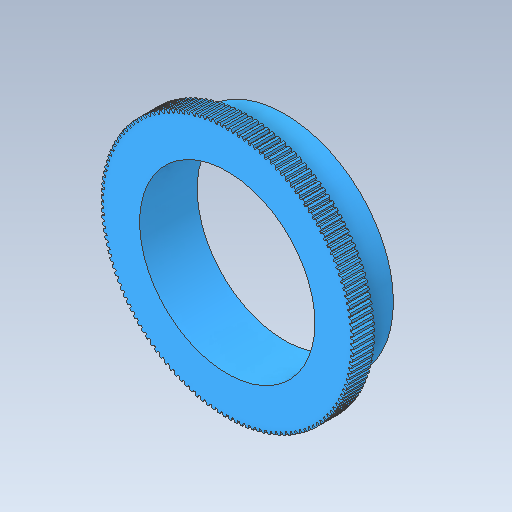
# Autodesk Inventor part: タミヤダンパー4
Saved by Autodesk Inventor 2020 (Build 240168000, 168)
## iProperties
Part Number: タミヤダンパー4
Material: 一般
Document SubType Name: Modeling
Designer: 雪村
Density: 1 g/cm^3
Appearance: 既定
Mass: 0.362407 g
Surface Area: 6.8095 cm^2
Volume: 0.362407 cm^3
Author: 雪村
Autodesk Inventor part; units mm, degrees
ref_plane "YZ Plane" through (0, 0, 0) normal (1, 0, 0) x (0, 1, 0)
ref_plane "XZ Plane" through (0, 0, 0) normal (0, 1, 0) x (-1, 0, 0)
ref_plane "XY Plane" through (0, 0, 0) normal (0, 0, 1) x (1, 0, 0)
sketch "スケッチ1" plane through (0, 0, 0) normal (0, 0, 1) x (1, 0, 0)
  circle A0 centre (0, 0) radius 7.75
  dimension "d0" = 15.5
  constraints: 1 centre point, 1 coincident
  measures "d0" diameter of A0
extrude "押し出し1" add sketch "スケッチ1" along normal blind 2.6
sketch "スケッチ2" plane through (0, 0, 2.6) normal (0, 0, 1) x (1, 0, 0)
  circle A0 centre (0, 0) radius 9
  dimension "d3" = 18
  constraints: 1 centre point, 1 coincident
  measures "d3" diameter of A0
extrude "押し出し2" add sketch "スケッチ2" along normal blind 1.5
sketch "スケッチ3" plane through (0, 0, 4.1) normal (0, 0, 1) x (1, 0, 0)
  circle A0 centre (0, 0) radius 6.25
  dimension "d6" = 12.5
  constraints: 1 centre point, 1 coincident
  measures "d6" diameter of A0
extrude "押し出し3" cut sketch "スケッチ3" against normal through all
sketch "スケッチ4" plane through (0, 0, 4.1) normal (0, 0, 1) x (1, 0, 0)
  arc A0 (-0.1214, -8.9992) -> (0.1214, -8.9992) centre (0, 0) ccw
  arc A1 (-0.05, -8.8124) -> (0.05, -8.8124) centre (0, 0) ccw
  line L0 (0.1214, -8.9992) -> (0.05, -8.8124)
  line L1 (-0.05, -8.8124) -> (-0.1214, -8.9992)
  line L2 (0, -8.8125) -> (0, 0)
  line L3 (0.525, -8.9847) -> (0.4453, -8.8012)
  arc A2 (0.2825, -8.9956) -> (0.525, -8.9847) centre (0, 0) ccw
  line L4 (0.3454, -8.8057) -> (0.2825, -8.9956)
  arc A3 (0.3454, -8.8057) -> (0.4453, -8.8012) centre (0, 0) ccw
  line L5 (0.9276, -8.9521) -> (0.8397, -8.7724)
  arc A4 (0.6858, -8.9738) -> (0.9276, -8.9521) centre (0, 0) ccw
  line L6 (0.7401, -8.7814) -> (0.6858, -8.9738)
  arc A5 (0.7401, -8.7814) -> (0.8397, -8.7724) centre (0, 0) ccw
  line L7 (1.3283, -8.9014) -> (1.2325, -8.7259)
  arc A6 (1.0877, -8.934) -> (1.3283, -8.9014) centre (0, 0) ccw
  line L8 (1.1334, -8.7393) -> (1.0877, -8.934)
  arc A7 (1.1334, -8.7393) -> (1.2325, -8.7259) centre (0, 0) ccw
  line L9 (1.7263, -8.8329) -> (1.6227, -8.6618)
  arc A8 (1.4874, -8.8762) -> (1.7263, -8.8329) centre (0, 0) ccw
  line L10 (1.5243, -8.6797) -> (1.4874, -8.8762)
  arc A9 (1.5243, -8.6797) -> (1.6227, -8.6618) centre (0, 0) ccw
  line L11 (2.1209, -8.7465) -> (2.0097, -8.5803)
  arc A10 (1.8842, -8.8006) -> (2.1209, -8.7465) centre (0, 0) ccw
  line L12 (1.9122, -8.6025) -> (1.8842, -8.8006)
  arc A11 (1.9122, -8.6025) -> (2.0097, -8.5803) centre (0, 0) ccw
  line L13 (2.5111, -8.6426) -> (2.3926, -8.4815)
  arc A12 (2.2771, -8.7072) -> (2.5111, -8.6426) centre (0, 0) ccw
  line L14 (2.2962, -8.5081) -> (2.2771, -8.7072)
  arc A13 (2.2962, -8.5081) -> (2.3926, -8.4815) centre (0, 0) ccw
  line L15 (2.8964, -8.5212) -> (2.7707, -8.3656)
  arc A14 (2.6654, -8.5962) -> (2.8964, -8.5212) centre (0, 0) ccw
  line L16 (2.6756, -8.3965) -> (2.6654, -8.5962)
  arc A15 (2.6756, -8.3965) -> (2.7707, -8.3656) centre (0, 0) ccw
  line L17 (3.2757, -8.3827) -> (3.1433, -8.2329)
  arc A16 (3.0484, -8.468) -> (3.2757, -8.3827) centre (0, 0) ccw
  line L18 (3.0496, -8.268) -> (3.0484, -8.468)
  arc A17 (3.0496, -8.268) -> (3.1433, -8.2329) centre (0, 0) ccw
  line L19 (3.6485, -8.2273) -> (3.5095, -8.0836)
  arc A18 (3.4253, -8.3227) -> (3.6485, -8.2273) centre (0, 0) ccw
  line L20 (3.4175, -8.1229) -> (3.4253, -8.3227)
  arc A19 (3.4175, -8.1229) -> (3.5095, -8.0836) centre (0, 0) ccw
  line L21 (4.014, -8.0553) -> (3.8686, -7.918)
  arc A20 (3.7952, -8.1607) -> (4.014, -8.0553) centre (0, 0) ccw
  line L22 (3.7785, -7.9614) -> (3.7952, -8.1607)
  arc A21 (3.7785, -7.9614) -> (3.8686, -7.918) centre (0, 0) ccw
  line L23 (4.3713, -7.8671) -> (4.2199, -7.7364)
  arc A22 (4.1575, -7.9822) -> (4.3713, -7.8671) centre (0, 0) ccw
  line L24 (4.1319, -7.7838) -> (4.1575, -7.9822)
  arc A23 (4.1319, -7.7838) -> (4.2199, -7.7364) centre (0, 0) ccw
  line L25 (4.7199, -7.6631) -> (4.5628, -7.5393)
  arc A24 (4.5115, -7.7876) -> (4.7199, -7.6631) centre (0, 0) ccw
  line L26 (4.4769, -7.5906) -> (4.5115, -7.7876)
  arc A25 (4.4769, -7.5906) -> (4.5628, -7.5393) centre (0, 0) ccw
  line L27 (5.0589, -7.4436) -> (4.8964, -7.327)
  arc A26 (4.8563, -7.5774) -> (5.0589, -7.4436) centre (0, 0) ccw
  line L28 (4.813, -7.3821) -> (4.8563, -7.5774)
  arc A27 (4.813, -7.3821) -> (4.8964, -7.327) centre (0, 0) ccw
  line L29 (5.3878, -7.2091) -> (5.2202, -7.1)
  arc A28 (5.1914, -7.3518) -> (5.3878, -7.2091) centre (0, 0) ccw
  line L30 (5.1393, -7.1587) -> (5.1914, -7.3518)
  arc A29 (5.1393, -7.1587) -> (5.2202, -7.1) centre (0, 0) ccw
  line L31 (5.7058, -6.9602) -> (5.5335, -6.8586)
  arc A30 (5.516, -7.1115) -> (5.7058, -6.9602) centre (0, 0) ccw
  line L32 (5.4553, -6.921) -> (5.516, -7.1115)
  arc A31 (5.4553, -6.921) -> (5.5335, -6.8586) centre (0, 0) ccw
  line L33 (6.0123, -6.6972) -> (5.8356, -6.6034)
  arc A32 (5.8295, -6.8569) -> (6.0123, -6.6972) centre (0, 0) ccw
  line L34 (5.7603, -6.6692) -> (5.8295, -6.8569)
  arc A33 (5.7603, -6.6692) -> (5.8356, -6.6034) centre (0, 0) ccw
  line L35 (6.3067, -6.4207) -> (6.126, -6.335)
  arc A34 (6.1313, -6.5885) -> (6.3067, -6.4207) centre (0, 0) ccw
  line L36 (6.0538, -6.4041) -> (6.1313, -6.5885)
  arc A35 (6.0538, -6.4041) -> (6.126, -6.335) centre (0, 0) ccw
  line L37 (6.5885, -6.1313) -> (6.4041, -6.0538)
  arc A36 (6.4207, -6.3067) -> (6.5885, -6.1313) centre (0, 0) ccw
  line L38 (6.335, -6.126) -> (6.4207, -6.3067)
  arc A37 (6.335, -6.126) -> (6.4041, -6.0538) centre (0, 0) ccw
  line L39 (6.8569, -5.8295) -> (6.6692, -5.7603)
  arc A38 (6.6972, -6.0123) -> (6.8569, -5.8295) centre (0, 0) ccw
  line L40 (6.6034, -5.8356) -> (6.6972, -6.0123)
  arc A39 (6.6034, -5.8356) -> (6.6692, -5.7603) centre (0, 0) ccw
  line L41 (7.1115, -5.516) -> (6.921, -5.4553)
  arc A40 (6.9602, -5.7058) -> (7.1115, -5.516) centre (0, 0) ccw
  line L42 (6.8586, -5.5335) -> (6.9602, -5.7058)
  arc A41 (6.8586, -5.5335) -> (6.921, -5.4553) centre (0, 0) ccw
  line L43 (7.3518, -5.1914) -> (7.1587, -5.1393)
  arc A42 (7.2091, -5.3878) -> (7.3518, -5.1914) centre (0, 0) ccw
  line L44 (7.1, -5.2202) -> (7.2091, -5.3878)
  arc A43 (7.1, -5.2202) -> (7.1587, -5.1393) centre (0, 0) ccw
  line L45 (7.5774, -4.8563) -> (7.3821, -4.813)
  arc A44 (7.4436, -5.0589) -> (7.5774, -4.8563) centre (0, 0) ccw
  line L46 (7.327, -4.8964) -> (7.4436, -5.0589)
  arc A45 (7.327, -4.8964) -> (7.3821, -4.813) centre (0, 0) ccw
  line L47 (7.7876, -4.5115) -> (7.5906, -4.4769)
  arc A46 (7.6631, -4.7199) -> (7.7876, -4.5115) centre (0, 0) ccw
  line L48 (7.5393, -4.5628) -> (7.6631, -4.7199)
  arc A47 (7.5393, -4.5628) -> (7.5906, -4.4769) centre (0, 0) ccw
  line L49 (7.9822, -4.1575) -> (7.7838, -4.1319)
  arc A48 (7.8671, -4.3713) -> (7.9822, -4.1575) centre (0, 0) ccw
  line L50 (7.7364, -4.2199) -> (7.8671, -4.3713)
  arc A49 (7.7364, -4.2199) -> (7.7838, -4.1319) centre (0, 0) ccw
  line L51 (8.1607, -3.7952) -> (7.9614, -3.7785)
  arc A50 (8.0553, -4.014) -> (8.1607, -3.7952) centre (0, 0) ccw
  line L52 (7.918, -3.8686) -> (8.0553, -4.014)
  arc A51 (7.918, -3.8686) -> (7.9614, -3.7785) centre (0, 0) ccw
  line L53 (8.3227, -3.4253) -> (8.1229, -3.4175)
  arc A52 (8.2273, -3.6485) -> (8.3227, -3.4253) centre (0, 0) ccw
  line L54 (8.0836, -3.5095) -> (8.2273, -3.6485)
  arc A53 (8.0836, -3.5095) -> (8.1229, -3.4175) centre (0, 0) ccw
  line L55 (8.468, -3.0484) -> (8.268, -3.0496)
  arc A54 (8.3827, -3.2757) -> (8.468, -3.0484) centre (0, 0) ccw
  line L56 (8.2329, -3.1433) -> (8.3827, -3.2757)
  arc A55 (8.2329, -3.1433) -> (8.268, -3.0496) centre (0, 0) ccw
  line L57 (8.5962, -2.6654) -> (8.3965, -2.6756)
  arc A56 (8.5212, -2.8964) -> (8.5962, -2.6654) centre (0, 0) ccw
  line L58 (8.3656, -2.7707) -> (8.5212, -2.8964)
  arc A57 (8.3656, -2.7707) -> (8.3965, -2.6756) centre (0, 0) ccw
  line L59 (8.7072, -2.2771) -> (8.5081, -2.2962)
  arc A58 (8.6426, -2.5111) -> (8.7072, -2.2771) centre (0, 0) ccw
  line L60 (8.4815, -2.3926) -> (8.6426, -2.5111)
  arc A59 (8.4815, -2.3926) -> (8.5081, -2.2962) centre (0, 0) ccw
  line L61 (8.8006, -1.8842) -> (8.6025, -1.9122)
  arc A60 (8.7465, -2.1209) -> (8.8006, -1.8842) centre (0, 0) ccw
  line L62 (8.5803, -2.0097) -> (8.7465, -2.1209)
  arc A61 (8.5803, -2.0097) -> (8.6025, -1.9122) centre (0, 0) ccw
  line L63 (8.8762, -1.4874) -> (8.6797, -1.5243)
  arc A62 (8.8329, -1.7263) -> (8.8762, -1.4874) centre (0, 0) ccw
  line L64 (8.6618, -1.6227) -> (8.8329, -1.7263)
  arc A63 (8.6618, -1.6227) -> (8.6797, -1.5243) centre (0, 0) ccw
  line L65 (8.934, -1.0877) -> (8.7393, -1.1334)
  arc A64 (8.9014, -1.3283) -> (8.934, -1.0877) centre (0, 0) ccw
  line L66 (8.7259, -1.2325) -> (8.9014, -1.3283)
  arc A65 (8.7259, -1.2325) -> (8.7393, -1.1334) centre (0, 0) ccw
  line L67 (8.9738, -0.6858) -> (8.7814, -0.7401)
  arc A66 (8.9521, -0.9276) -> (8.9738, -0.6858) centre (0, 0) ccw
  line L68 (8.7724, -0.8397) -> (8.9521, -0.9276)
  arc A67 (8.7724, -0.8397) -> (8.7814, -0.7401) centre (0, 0) ccw
  line L69 (8.9956, -0.2825) -> (8.8057, -0.3454)
  arc A68 (8.9847, -0.525) -> (8.9956, -0.2825) centre (0, 0) ccw
  line L70 (8.8012, -0.4453) -> (8.9847, -0.525)
  arc A69 (8.8012, -0.4453) -> (8.8057, -0.3454) centre (0, 0) ccw
  line L71 (8.9992, 0.1214) -> (8.8124, 0.05)
  arc A70 (8.9992, -0.1214) -> (8.9992, 0.1214) centre (0, 0) ccw
  line L72 (8.8124, -0.05) -> (8.9992, -0.1214)
  arc A71 (8.8124, -0.05) -> (8.8124, 0.05) centre (0, 0) ccw
  line L73 (8.9847, 0.525) -> (8.8012, 0.4453)
  arc A72 (8.9956, 0.2825) -> (8.9847, 0.525) centre (0, 0) ccw
  line L74 (8.8057, 0.3454) -> (8.9956, 0.2825)
  arc A73 (8.8057, 0.3454) -> (8.8012, 0.4453) centre (0, 0) ccw
  line L75 (8.9521, 0.9276) -> (8.7724, 0.8397)
  arc A74 (8.9738, 0.6858) -> (8.9521, 0.9276) centre (0, 0) ccw
  line L76 (8.7814, 0.7401) -> (8.9738, 0.6858)
  arc A75 (8.7814, 0.7401) -> (8.7724, 0.8397) centre (0, 0) ccw
  line L77 (8.9014, 1.3283) -> (8.7259, 1.2325)
  arc A76 (8.934, 1.0877) -> (8.9014, 1.3283) centre (0, 0) ccw
  line L78 (8.7393, 1.1334) -> (8.934, 1.0877)
  arc A77 (8.7393, 1.1334) -> (8.7259, 1.2325) centre (0, 0) ccw
  line L79 (8.8329, 1.7263) -> (8.6618, 1.6227)
  arc A78 (8.8762, 1.4874) -> (8.8329, 1.7263) centre (0, 0) ccw
  line L80 (8.6797, 1.5243) -> (8.8762, 1.4874)
  arc A79 (8.6797, 1.5243) -> (8.6618, 1.6227) centre (0, 0) ccw
  line L81 (8.7465, 2.1209) -> (8.5803, 2.0097)
  arc A80 (8.8006, 1.8842) -> (8.7465, 2.1209) centre (0, 0) ccw
  line L82 (8.6025, 1.9122) -> (8.8006, 1.8842)
  arc A81 (8.6025, 1.9122) -> (8.5803, 2.0097) centre (0, 0) ccw
  line L83 (8.6426, 2.5111) -> (8.4815, 2.3926)
  arc A82 (8.7072, 2.2771) -> (8.6426, 2.5111) centre (0, 0) ccw
  line L84 (8.5081, 2.2962) -> (8.7072, 2.2771)
  arc A83 (8.5081, 2.2962) -> (8.4815, 2.3926) centre (0, 0) ccw
  line L85 (8.5212, 2.8964) -> (8.3656, 2.7707)
  arc A84 (8.5962, 2.6654) -> (8.5212, 2.8964) centre (0, 0) ccw
  line L86 (8.3965, 2.6756) -> (8.5962, 2.6654)
  arc A85 (8.3965, 2.6756) -> (8.3656, 2.7707) centre (0, 0) ccw
  line L87 (8.3827, 3.2757) -> (8.2329, 3.1433)
  arc A86 (8.468, 3.0484) -> (8.3827, 3.2757) centre (0, 0) ccw
  line L88 (8.268, 3.0496) -> (8.468, 3.0484)
  arc A87 (8.268, 3.0496) -> (8.2329, 3.1433) centre (0, 0) ccw
  line L89 (8.2273, 3.6485) -> (8.0836, 3.5095)
  arc A88 (8.3227, 3.4253) -> (8.2273, 3.6485) centre (0, 0) ccw
  line L90 (8.1229, 3.4175) -> (8.3227, 3.4253)
  arc A89 (8.1229, 3.4175) -> (8.0836, 3.5095) centre (0, 0) ccw
  line L91 (8.0553, 4.014) -> (7.918, 3.8686)
  arc A90 (8.1607, 3.7952) -> (8.0553, 4.014) centre (0, 0) ccw
  line L92 (7.9614, 3.7785) -> (8.1607, 3.7952)
  arc A91 (7.9614, 3.7785) -> (7.918, 3.8686) centre (0, 0) ccw
  line L93 (7.8671, 4.3713) -> (7.7364, 4.2199)
  arc A92 (7.9822, 4.1575) -> (7.8671, 4.3713) centre (0, 0) ccw
  line L94 (7.7838, 4.1319) -> (7.9822, 4.1575)
  arc A93 (7.7838, 4.1319) -> (7.7364, 4.2199) centre (0, 0) ccw
  line L95 (7.6631, 4.7199) -> (7.5393, 4.5628)
  arc A94 (7.7876, 4.5115) -> (7.6631, 4.7199) centre (0, 0) ccw
  line L96 (7.5906, 4.4769) -> (7.7876, 4.5115)
  arc A95 (7.5906, 4.4769) -> (7.5393, 4.5628) centre (0, 0) ccw
  line L97 (7.4436, 5.0589) -> (7.327, 4.8964)
  arc A96 (7.5774, 4.8563) -> (7.4436, 5.0589) centre (0, 0) ccw
  line L98 (7.3821, 4.813) -> (7.5774, 4.8563)
  arc A97 (7.3821, 4.813) -> (7.327, 4.8964) centre (0, 0) ccw
  line L99 (7.2091, 5.3878) -> (7.1, 5.2202)
  arc A98 (7.3518, 5.1914) -> (7.2091, 5.3878) centre (0, 0) ccw
  line L100 (7.1587, 5.1393) -> (7.3518, 5.1914)
  arc A99 (7.1587, 5.1393) -> (7.1, 5.2202) centre (0, 0) ccw
  line L101 (6.9602, 5.7058) -> (6.8586, 5.5335)
  arc A100 (7.1115, 5.516) -> (6.9602, 5.7058) centre (0, 0) ccw
  line L102 (6.921, 5.4553) -> (7.1115, 5.516)
  arc A101 (6.921, 5.4553) -> (6.8586, 5.5335) centre (0, 0) ccw
  line L103 (6.6972, 6.0123) -> (6.6034, 5.8356)
  arc A102 (6.8569, 5.8295) -> (6.6972, 6.0123) centre (0, 0) ccw
  line L104 (6.6692, 5.7603) -> (6.8569, 5.8295)
  arc A103 (6.6692, 5.7603) -> (6.6034, 5.8356) centre (0, 0) ccw
  line L105 (6.4207, 6.3067) -> (6.335, 6.126)
  arc A104 (6.5885, 6.1313) -> (6.4207, 6.3067) centre (0, 0) ccw
  line L106 (6.4041, 6.0538) -> (6.5885, 6.1313)
  arc A105 (6.4041, 6.0538) -> (6.335, 6.126) centre (0, 0) ccw
  line L107 (6.1313, 6.5885) -> (6.0538, 6.4041)
  arc A106 (6.3067, 6.4207) -> (6.1313, 6.5885) centre (0, 0) ccw
  line L108 (6.126, 6.335) -> (6.3067, 6.4207)
  arc A107 (6.126, 6.335) -> (6.0538, 6.4041) centre (0, 0) ccw
  line L109 (5.8295, 6.8569) -> (5.7603, 6.6692)
  arc A108 (6.0123, 6.6972) -> (5.8295, 6.8569) centre (0, 0) ccw
  line L110 (5.8356, 6.6034) -> (6.0123, 6.6972)
  arc A109 (5.8356, 6.6034) -> (5.7603, 6.6692) centre (0, 0) ccw
  line L111 (5.516, 7.1115) -> (5.4553, 6.921)
  arc A110 (5.7058, 6.9602) -> (5.516, 7.1115) centre (0, 0) ccw
  line L112 (5.5335, 6.8586) -> (5.7058, 6.9602)
  arc A111 (5.5335, 6.8586) -> (5.4553, 6.921) centre (0, 0) ccw
  line L113 (5.1914, 7.3518) -> (5.1393, 7.1587)
  arc A112 (5.3878, 7.2091) -> (5.1914, 7.3518) centre (0, 0) ccw
  line L114 (5.2202, 7.1) -> (5.3878, 7.2091)
  arc A113 (5.2202, 7.1) -> (5.1393, 7.1587) centre (0, 0) ccw
  line L115 (4.8563, 7.5774) -> (4.813, 7.3821)
  arc A114 (5.0589, 7.4436) -> (4.8563, 7.5774) centre (0, 0) ccw
  line L116 (4.8964, 7.327) -> (5.0589, 7.4436)
  arc A115 (4.8964, 7.327) -> (4.813, 7.3821) centre (0, 0) ccw
  line L117 (4.5115, 7.7876) -> (4.4769, 7.5906)
  arc A116 (4.7199, 7.6631) -> (4.5115, 7.7876) centre (0, 0) ccw
  line L118 (4.5628, 7.5393) -> (4.7199, 7.6631)
  arc A117 (4.5628, 7.5393) -> (4.4769, 7.5906) centre (0, 0) ccw
  line L119 (4.1575, 7.9822) -> (4.1319, 7.7838)
  arc A118 (4.3713, 7.8671) -> (4.1575, 7.9822) centre (0, 0) ccw
  line L120 (4.2199, 7.7364) -> (4.3713, 7.8671)
  arc A119 (4.2199, 7.7364) -> (4.1319, 7.7838) centre (0, 0) ccw
  line L121 (3.7952, 8.1607) -> (3.7785, 7.9614)
  arc A120 (4.014, 8.0553) -> (3.7952, 8.1607) centre (0, 0) ccw
  line L122 (3.8686, 7.918) -> (4.014, 8.0553)
  arc A121 (3.8686, 7.918) -> (3.7785, 7.9614) centre (0, 0) ccw
  line L123 (3.4253, 8.3227) -> (3.4175, 8.1229)
  arc A122 (3.6485, 8.2273) -> (3.4253, 8.3227) centre (0, 0) ccw
  line L124 (3.5095, 8.0836) -> (3.6485, 8.2273)
  arc A123 (3.5095, 8.0836) -> (3.4175, 8.1229) centre (0, 0) ccw
  line L125 (3.0484, 8.468) -> (3.0496, 8.268)
  arc A124 (3.2757, 8.3827) -> (3.0484, 8.468) centre (0, 0) ccw
  line L126 (3.1433, 8.2329) -> (3.2757, 8.3827)
  arc A125 (3.1433, 8.2329) -> (3.0496, 8.268) centre (0, 0) ccw
  line L127 (2.6654, 8.5962) -> (2.6756, 8.3965)
  arc A126 (2.8964, 8.5212) -> (2.6654, 8.5962) centre (0, 0) ccw
  line L128 (2.7707, 8.3656) -> (2.8964, 8.5212)
  arc A127 (2.7707, 8.3656) -> (2.6756, 8.3965) centre (0, 0) ccw
  line L129 (2.2771, 8.7072) -> (2.2962, 8.5081)
  arc A128 (2.5111, 8.6426) -> (2.2771, 8.7072) centre (0, 0) ccw
  line L130 (2.3926, 8.4815) -> (2.5111, 8.6426)
  arc A129 (2.3926, 8.4815) -> (2.2962, 8.5081) centre (0, 0) ccw
  line L131 (1.8842, 8.8006) -> (1.9122, 8.6025)
  arc A130 (2.1209, 8.7465) -> (1.8842, 8.8006) centre (0, 0) ccw
  line L132 (2.0097, 8.5803) -> (2.1209, 8.7465)
  arc A131 (2.0097, 8.5803) -> (1.9122, 8.6025) centre (0, 0) ccw
  line L133 (1.4874, 8.8762) -> (1.5243, 8.6797)
  arc A132 (1.7263, 8.8329) -> (1.4874, 8.8762) centre (0, 0) ccw
  line L134 (1.6227, 8.6618) -> (1.7263, 8.8329)
  arc A133 (1.6227, 8.6618) -> (1.5243, 8.6797) centre (0, 0) ccw
  line L135 (1.0877, 8.934) -> (1.1334, 8.7393)
  arc A134 (1.3283, 8.9014) -> (1.0877, 8.934) centre (0, 0) ccw
  line L136 (1.2325, 8.7259) -> (1.3283, 8.9014)
  arc A135 (1.2325, 8.7259) -> (1.1334, 8.7393) centre (0, 0) ccw
  line L137 (0.6858, 8.9738) -> (0.7401, 8.7814)
  arc A136 (0.9276, 8.9521) -> (0.6858, 8.9738) centre (0, 0) ccw
  line L138 (0.8397, 8.7724) -> (0.9276, 8.9521)
  arc A137 (0.8397, 8.7724) -> (0.7401, 8.7814) centre (0, 0) ccw
  line L139 (0.2825, 8.9956) -> (0.3454, 8.8057)
  arc A138 (0.525, 8.9847) -> (0.2825, 8.9956) centre (0, 0) ccw
  line L140 (0.4453, 8.8012) -> (0.525, 8.9847)
  arc A139 (0.4453, 8.8012) -> (0.3454, 8.8057) centre (0, 0) ccw
  line L141 (-0.1214, 8.9992) -> (-0.05, 8.8124)
  arc A140 (0.1214, 8.9992) -> (-0.1214, 8.9992) centre (0, 0) ccw
  line L142 (0.05, 8.8124) -> (0.1214, 8.9992)
  arc A141 (0.05, 8.8124) -> (-0.05, 8.8124) centre (0, 0) ccw
  line L143 (-0.525, 8.9847) -> (-0.4453, 8.8012)
  arc A142 (-0.2825, 8.9956) -> (-0.525, 8.9847) centre (0, 0) ccw
  line L144 (-0.3454, 8.8057) -> (-0.2825, 8.9956)
  arc A143 (-0.3454, 8.8057) -> (-0.4453, 8.8012) centre (0, 0) ccw
  line L145 (-0.9276, 8.9521) -> (-0.8397, 8.7724)
  arc A144 (-0.6858, 8.9738) -> (-0.9276, 8.9521) centre (0, 0) ccw
  line L146 (-0.7401, 8.7814) -> (-0.6858, 8.9738)
  arc A145 (-0.7401, 8.7814) -> (-0.8397, 8.7724) centre (0, 0) ccw
  line L147 (-1.3283, 8.9014) -> (-1.2325, 8.7259)
  arc A146 (-1.0877, 8.934) -> (-1.3283, 8.9014) centre (0, 0) ccw
  line L148 (-1.1334, 8.7393) -> (-1.0877, 8.934)
  arc A147 (-1.1334, 8.7393) -> (-1.2325, 8.7259) centre (0, 0) ccw
  line L149 (-1.7263, 8.8329) -> (-1.6227, 8.6618)
  arc A148 (-1.4874, 8.8762) -> (-1.7263, 8.8329) centre (0, 0) ccw
  line L150 (-1.5243, 8.6797) -> (-1.4874, 8.8762)
  arc A149 (-1.5243, 8.6797) -> (-1.6227, 8.6618) centre (0, 0) ccw
  line L151 (-2.1209, 8.7465) -> (-2.0097, 8.5803)
  arc A150 (-1.8842, 8.8006) -> (-2.1209, 8.7465) centre (0, 0) ccw
  line L152 (-1.9122, 8.6025) -> (-1.8842, 8.8006)
  arc A151 (-1.9122, 8.6025) -> (-2.0097, 8.5803) centre (0, 0) ccw
  line L153 (-2.5111, 8.6426) -> (-2.3926, 8.4815)
  arc A152 (-2.2771, 8.7072) -> (-2.5111, 8.6426) centre (0, 0) ccw
  line L154 (-2.2962, 8.5081) -> (-2.2771, 8.7072)
  arc A153 (-2.2962, 8.5081) -> (-2.3926, 8.4815) centre (0, 0) ccw
  line L155 (-2.8964, 8.5212) -> (-2.7707, 8.3656)
  arc A154 (-2.6654, 8.5962) -> (-2.8964, 8.5212) centre (0, 0) ccw
  line L156 (-2.6756, 8.3965) -> (-2.6654, 8.5962)
  arc A155 (-2.6756, 8.3965) -> (-2.7707, 8.3656) centre (0, 0) ccw
  line L157 (-3.2757, 8.3827) -> (-3.1433, 8.2329)
  arc A156 (-3.0484, 8.468) -> (-3.2757, 8.3827) centre (0, 0) ccw
  line L158 (-3.0496, 8.268) -> (-3.0484, 8.468)
  arc A157 (-3.0496, 8.268) -> (-3.1433, 8.2329) centre (0, 0) ccw
  line L159 (-3.6485, 8.2273) -> (-3.5095, 8.0836)
  arc A158 (-3.4253, 8.3227) -> (-3.6485, 8.2273) centre (0, 0) ccw
  line L160 (-3.4175, 8.1229) -> (-3.4253, 8.3227)
  arc A159 (-3.4175, 8.1229) -> (-3.5095, 8.0836) centre (0, 0) ccw
  line L161 (-4.014, 8.0553) -> (-3.8686, 7.918)
  arc A160 (-3.7952, 8.1607) -> (-4.014, 8.0553) centre (0, 0) ccw
  line L162 (-3.7785, 7.9614) -> (-3.7952, 8.1607)
  arc A161 (-3.7785, 7.9614) -> (-3.8686, 7.918) centre (0, 0) ccw
  line L163 (-4.3713, 7.8671) -> (-4.2199, 7.7364)
  arc A162 (-4.1575, 7.9822) -> (-4.3713, 7.8671) centre (0, 0) ccw
  line L164 (-4.1319, 7.7838) -> (-4.1575, 7.9822)
  arc A163 (-4.1319, 7.7838) -> (-4.2199, 7.7364) centre (0, 0) ccw
  line L165 (-4.7199, 7.6631) -> (-4.5628, 7.5393)
  arc A164 (-4.5115, 7.7876) -> (-4.7199, 7.6631) centre (0, 0) ccw
  line L166 (-4.4769, 7.5906) -> (-4.5115, 7.7876)
  arc A165 (-4.4769, 7.5906) -> (-4.5628, 7.5393) centre (0, 0) ccw
  line L167 (-5.0589, 7.4436) -> (-4.8964, 7.327)
  arc A166 (-4.8563, 7.5774) -> (-5.0589, 7.4436) centre (0, 0) ccw
  line L168 (-4.813, 7.3821) -> (-4.8563, 7.5774)
  arc A167 (-4.813, 7.3821) -> (-4.8964, 7.327) centre (0, 0) ccw
  line L169 (-5.3878, 7.2091) -> (-5.2202, 7.1)
  arc A168 (-5.1914, 7.3518) -> (-5.3878, 7.2091) centre (0, 0) ccw
  line L170 (-5.1393, 7.1587) -> (-5.1914, 7.3518)
  arc A169 (-5.1393, 7.1587) -> (-5.2202, 7.1) centre (0, 0) ccw
  line L171 (-5.7058, 6.9602) -> (-5.5335, 6.8586)
  arc A170 (-5.516, 7.1115) -> (-5.7058, 6.9602) centre (0, 0) ccw
  line L172 (-5.4553, 6.921) -> (-5.516, 7.1115)
  arc A171 (-5.4553, 6.921) -> (-5.5335, 6.8586) centre (0, 0) ccw
  line L173 (-6.0123, 6.6972) -> (-5.8356, 6.6034)
  arc A172 (-5.8295, 6.8569) -> (-6.0123, 6.6972) centre (0, 0) ccw
  line L174 (-5.7603, 6.6692) -> (-5.8295, 6.8569)
  arc A173 (-5.7603, 6.6692) -> (-5.8356, 6.6034) centre (0, 0) ccw
  line L175 (-6.3067, 6.4207) -> (-6.126, 6.335)
  arc A174 (-6.1313, 6.5885) -> (-6.3067, 6.4207) centre (0, 0) ccw
  line L176 (-6.0538, 6.4041) -> (-6.1313, 6.5885)
  arc A175 (-6.0538, 6.4041) -> (-6.126, 6.335) centre (0, 0) ccw
  line L177 (-6.5885, 6.1313) -> (-6.4041, 6.0538)
  arc A176 (-6.4207, 6.3067) -> (-6.5885, 6.1313) centre (0, 0) ccw
  line L178 (-6.335, 6.126) -> (-6.4207, 6.3067)
  arc A177 (-6.335, 6.126) -> (-6.4041, 6.0538) centre (0, 0) ccw
  line L179 (-6.8569, 5.8295) -> (-6.6692, 5.7603)
  arc A178 (-6.6972, 6.0123) -> (-6.8569, 5.8295) centre (0, 0) ccw
  line L180 (-6.6034, 5.8356) -> (-6.6972, 6.0123)
  arc A179 (-6.6034, 5.8356) -> (-6.6692, 5.7603) centre (0, 0) ccw
  line L181 (-7.1115, 5.516) -> (-6.921, 5.4553)
  arc A180 (-6.9602, 5.7058) -> (-7.1115, 5.516) centre (0, 0) ccw
  line L182 (-6.8586, 5.5335) -> (-6.9602, 5.7058)
  arc A181 (-6.8586, 5.5335) -> (-6.921, 5.4553) centre (0, 0) ccw
  line L183 (-7.3518, 5.1914) -> (-7.1587, 5.1393)
  arc A182 (-7.2091, 5.3878) -> (-7.3518, 5.1914) centre (0, 0) ccw
  line L184 (-7.1, 5.2202) -> (-7.2091, 5.3878)
  arc A183 (-7.1, 5.2202) -> (-7.1587, 5.1393) centre (0, 0) ccw
  line L185 (-7.5774, 4.8563) -> (-7.3821, 4.813)
  arc A184 (-7.4436, 5.0589) -> (-7.5774, 4.8563) centre (0, 0) ccw
  line L186 (-7.327, 4.8964) -> (-7.4436, 5.0589)
  arc A185 (-7.327, 4.8964) -> (-7.3821, 4.813) centre (0, 0) ccw
  line L187 (-7.7876, 4.5115) -> (-7.5906, 4.4769)
  arc A186 (-7.6631, 4.7199) -> (-7.7876, 4.5115) centre (0, 0) ccw
  line L188 (-7.5393, 4.5628) -> (-7.6631, 4.7199)
  arc A187 (-7.5393, 4.5628) -> (-7.5906, 4.4769) centre (0, 0) ccw
  line L189 (-7.9822, 4.1575) -> (-7.7838, 4.1319)
  arc A188 (-7.8671, 4.3713) -> (-7.9822, 4.1575) centre (0, 0) ccw
  line L190 (-7.7364, 4.2199) -> (-7.8671, 4.3713)
  arc A189 (-7.7364, 4.2199) -> (-7.7838, 4.1319) centre (0, 0) ccw
  line L191 (-8.1607, 3.7952) -> (-7.9614, 3.7785)
  arc A190 (-8.0553, 4.014) -> (-8.1607, 3.7952) centre (0, 0) ccw
  line L192 (-7.918, 3.8686) -> (-8.0553, 4.014)
  arc A191 (-7.918, 3.8686) -> (-7.9614, 3.7785) centre (0, 0) ccw
  line L193 (-8.3227, 3.4253) -> (-8.1229, 3.4175)
  arc A192 (-8.2273, 3.6485) -> (-8.3227, 3.4253) centre (0, 0) ccw
  line L194 (-8.0836, 3.5095) -> (-8.2273, 3.6485)
  arc A193 (-8.0836, 3.5095) -> (-8.1229, 3.4175) centre (0, 0) ccw
  line L195 (-8.468, 3.0484) -> (-8.268, 3.0496)
  arc A194 (-8.3827, 3.2757) -> (-8.468, 3.0484) centre (0, 0) ccw
  line L196 (-8.2329, 3.1433) -> (-8.3827, 3.2757)
  arc A195 (-8.2329, 3.1433) -> (-8.268, 3.0496) centre (0, 0) ccw
  line L197 (-8.5962, 2.6654) -> (-8.3965, 2.6756)
  arc A196 (-8.5212, 2.8964) -> (-8.5962, 2.6654) centre (0, 0) ccw
  line L198 (-8.3656, 2.7707) -> (-8.5212, 2.8964)
  arc A197 (-8.3656, 2.7707) -> (-8.3965, 2.6756) centre (0, 0) ccw
  line L199 (-8.7072, 2.2771) -> (-8.5081, 2.2962)
  arc A198 (-8.6426, 2.5111) -> (-8.7072, 2.2771) centre (0, 0) ccw
  line L200 (-8.4815, 2.3926) -> (-8.6426, 2.5111)
  arc A199 (-8.4815, 2.3926) -> (-8.5081, 2.2962) centre (0, 0) ccw
  line L201 (-8.8006, 1.8842) -> (-8.6025, 1.9122)
  arc A200 (-8.7465, 2.1209) -> (-8.8006, 1.8842) centre (0, 0) ccw
  line L202 (-8.5803, 2.0097) -> (-8.7465, 2.1209)
  arc A201 (-8.5803, 2.0097) -> (-8.6025, 1.9122) centre (0, 0) ccw
  line L203 (-8.8762, 1.4874) -> (-8.6797, 1.5243)
  arc A202 (-8.8329, 1.7263) -> (-8.8762, 1.4874) centre (0, 0) ccw
  line L204 (-8.6618, 1.6227) -> (-8.8329, 1.7263)
  arc A203 (-8.6618, 1.6227) -> (-8.6797, 1.5243) centre (0, 0) ccw
  line L205 (-8.934, 1.0877) -> (-8.7393, 1.1334)
  arc A204 (-8.9014, 1.3283) -> (-8.934, 1.0877) centre (0, 0) ccw
  line L206 (-8.7259, 1.2325) -> (-8.9014, 1.3283)
  arc A205 (-8.7259, 1.2325) -> (-8.7393, 1.1334) centre (0, 0) ccw
  line L207 (-8.9738, 0.6858) -> (-8.7814, 0.7401)
  arc A206 (-8.9521, 0.9276) -> (-8.9738, 0.6858) centre (0, 0) ccw
  line L208 (-8.7724, 0.8397) -> (-8.9521, 0.9276)
  arc A207 (-8.7724, 0.8397) -> (-8.7814, 0.7401) centre (0, 0) ccw
  line L209 (-8.9956, 0.2825) -> (-8.8057, 0.3454)
  arc A208 (-8.9847, 0.525) -> (-8.9956, 0.2825) centre (0, 0) ccw
  line L210 (-8.8012, 0.4453) -> (-8.9847, 0.525)
  arc A209 (-8.8012, 0.4453) -> (-8.8057, 0.3454) centre (0, 0) ccw
  line L211 (-8.9992, -0.1214) -> (-8.8124, -0.05)
  arc A210 (-8.9992, 0.1214) -> (-8.9992, -0.1214) centre (0, 0) ccw
  line L212 (-8.8124, 0.05) -> (-8.9992, 0.1214)
  arc A211 (-8.8124, 0.05) -> (-8.8124, -0.05) centre (0, 0) ccw
  line L213 (-8.9847, -0.525) -> (-8.8012, -0.4453)
  arc A212 (-8.9956, -0.2825) -> (-8.9847, -0.525) centre (0, 0) ccw
  line L214 (-8.8057, -0.3454) -> (-8.9956, -0.2825)
  arc A213 (-8.8057, -0.3454) -> (-8.8012, -0.4453) centre (0, 0) ccw
  line L215 (-8.9521, -0.9276) -> (-8.7724, -0.8397)
  arc A214 (-8.9738, -0.6858) -> (-8.9521, -0.9276) centre (0, 0) ccw
  line L216 (-8.7814, -0.7401) -> (-8.9738, -0.6858)
  arc A215 (-8.7814, -0.7401) -> (-8.7724, -0.8397) centre (0, 0) ccw
  line L217 (-8.9014, -1.3283) -> (-8.7259, -1.2325)
  arc A216 (-8.934, -1.0877) -> (-8.9014, -1.3283) centre (0, 0) ccw
  line L218 (-8.7393, -1.1334) -> (-8.934, -1.0877)
  arc A217 (-8.7393, -1.1334) -> (-8.7259, -1.2325) centre (0, 0) ccw
  line L219 (-8.8329, -1.7263) -> (-8.6618, -1.6227)
  arc A218 (-8.8762, -1.4874) -> (-8.8329, -1.7263) centre (0, 0) ccw
  line L220 (-8.6797, -1.5243) -> (-8.8762, -1.4874)
  arc A219 (-8.6797, -1.5243) -> (-8.6618, -1.6227) centre (0, 0) ccw
  line L221 (-8.7465, -2.1209) -> (-8.5803, -2.0097)
  arc A220 (-8.8006, -1.8842) -> (-8.7465, -2.1209) centre (0, 0) ccw
  line L222 (-8.6025, -1.9122) -> (-8.8006, -1.8842)
  arc A221 (-8.6025, -1.9122) -> (-8.5803, -2.0097) centre (0, 0) ccw
  line L223 (-8.6426, -2.5111) -> (-8.4815, -2.3926)
  arc A222 (-8.7072, -2.2771) -> (-8.6426, -2.5111) centre (0, 0) ccw
  line L224 (-8.5081, -2.2962) -> (-8.7072, -2.2771)
  arc A223 (-8.5081, -2.2962) -> (-8.4815, -2.3926) centre (0, 0) ccw
  line L225 (-8.5212, -2.8964) -> (-8.3656, -2.7707)
  arc A224 (-8.5962, -2.6654) -> (-8.5212, -2.8964) centre (0, 0) ccw
  line L226 (-8.3965, -2.6756) -> (-8.5962, -2.6654)
  arc A225 (-8.3965, -2.6756) -> (-8.3656, -2.7707) centre (0, 0) ccw
  line L227 (-8.3827, -3.2757) -> (-8.2329, -3.1433)
  arc A226 (-8.468, -3.0484) -> (-8.3827, -3.2757) centre (0, 0) ccw
  line L228 (-8.268, -3.0496) -> (-8.468, -3.0484)
  arc A227 (-8.268, -3.0496) -> (-8.2329, -3.1433) centre (0, 0) ccw
  line L229 (-8.2273, -3.6485) -> (-8.0836, -3.5095)
  arc A228 (-8.3227, -3.4253) -> (-8.2273, -3.6485) centre (0, 0) ccw
  line L230 (-8.1229, -3.4175) -> (-8.3227, -3.4253)
  arc A229 (-8.1229, -3.4175) -> (-8.0836, -3.5095) centre (0, 0) ccw
  line L231 (-8.0553, -4.014) -> (-7.918, -3.8686)
  arc A230 (-8.1607, -3.7952) -> (-8.0553, -4.014) centre (0, 0) ccw
  line L232 (-7.9614, -3.7785) -> (-8.1607, -3.7952)
  arc A231 (-7.9614, -3.7785) -> (-7.918, -3.8686) centre (0, 0) ccw
  line L233 (-7.8671, -4.3713) -> (-7.7364, -4.2199)
  arc A232 (-7.9822, -4.1575) -> (-7.8671, -4.3713) centre (0, 0) ccw
  line L234 (-7.7838, -4.1319) -> (-7.9822, -4.1575)
  arc A233 (-7.7838, -4.1319) -> (-7.7364, -4.2199) centre (0, 0) ccw
  line L235 (-7.6631, -4.7199) -> (-7.5393, -4.5628)
  arc A234 (-7.7876, -4.5115) -> (-7.6631, -4.7199) centre (0, 0) ccw
  line L236 (-7.5906, -4.4769) -> (-7.7876, -4.5115)
  arc A235 (-7.5906, -4.4769) -> (-7.5393, -4.5628) centre (0, 0) ccw
  line L237 (-7.4436, -5.0589) -> (-7.327, -4.8964)
  arc A236 (-7.5774, -4.8563) -> (-7.4436, -5.0589) centre (0, 0) ccw
  line L238 (-7.3821, -4.813) -> (-7.5774, -4.8563)
  arc A237 (-7.3821, -4.813) -> (-7.327, -4.8964) centre (0, 0) ccw
  line L239 (-7.2091, -5.3878) -> (-7.1, -5.2202)
  arc A238 (-7.3518, -5.1914) -> (-7.2091, -5.3878) centre (0, 0) ccw
  line L240 (-7.1587, -5.1393) -> (-7.3518, -5.1914)
  arc A239 (-7.1587, -5.1393) -> (-7.1, -5.2202) centre (0, 0) ccw
  line L241 (-6.9602, -5.7058) -> (-6.8586, -5.5335)
  arc A240 (-7.1115, -5.516) -> (-6.9602, -5.7058) centre (0, 0) ccw
  line L242 (-6.921, -5.4553) -> (-7.1115, -5.516)
  arc A241 (-6.921, -5.4553) -> (-6.8586, -5.5335) centre (0, 0) ccw
  line L243 (-6.6972, -6.0123) -> (-6.6034, -5.8356)
  arc A242 (-6.8569, -5.8295) -> (-6.6972, -6.0123) centre (0, 0) ccw
  line L244 (-6.6692, -5.7603) -> (-6.8569, -5.8295)
  arc A243 (-6.6692, -5.7603) -> (-6.6034, -5.8356) centre (0, 0) ccw
  line L245 (-6.4207, -6.3067) -> (-6.335, -6.126)
  arc A244 (-6.5885, -6.1313) -> (-6.4207, -6.3067) centre (0, 0) ccw
  line L246 (-6.4041, -6.0538) -> (-6.5885, -6.1313)
  arc A245 (-6.4041, -6.0538) -> (-6.335, -6.126) centre (0, 0) ccw
  line L247 (-6.1313, -6.5885) -> (-6.0538, -6.4041)
  arc A246 (-6.3067, -6.4207) -> (-6.1313, -6.5885) centre (0, 0) ccw
  line L248 (-6.126, -6.335) -> (-6.3067, -6.4207)
  arc A247 (-6.126, -6.335) -> (-6.0538, -6.4041) centre (0, 0) ccw
  line L249 (-5.8295, -6.8569) -> (-5.7603, -6.6692)
  arc A248 (-6.0123, -6.6972) -> (-5.8295, -6.8569) centre (0, 0) ccw
  line L250 (-5.8356, -6.6034) -> (-6.0123, -6.6972)
  arc A249 (-5.8356, -6.6034) -> (-5.7603, -6.6692) centre (0, 0) ccw
  line L251 (-5.516, -7.1115) -> (-5.4553, -6.921)
  arc A250 (-5.7058, -6.9602) -> (-5.516, -7.1115) centre (0, 0) ccw
  line L252 (-5.5335, -6.8586) -> (-5.7058, -6.9602)
  arc A251 (-5.5335, -6.8586) -> (-5.4553, -6.921) centre (0, 0) ccw
  line L253 (-5.1914, -7.3518) -> (-5.1393, -7.1587)
  arc A252 (-5.3878, -7.2091) -> (-5.1914, -7.3518) centre (0, 0) ccw
  line L254 (-5.2202, -7.1) -> (-5.3878, -7.2091)
  arc A253 (-5.2202, -7.1) -> (-5.1393, -7.1587) centre (0, 0) ccw
  line L255 (-4.8563, -7.5774) -> (-4.813, -7.3821)
  arc A254 (-5.0589, -7.4436) -> (-4.8563, -7.5774) centre (0, 0) ccw
  line L256 (-4.8964, -7.327) -> (-5.0589, -7.4436)
  arc A255 (-4.8964, -7.327) -> (-4.813, -7.3821) centre (0, 0) ccw
  line L257 (-4.5115, -7.7876) -> (-4.4769, -7.5906)
  arc A256 (-4.7199, -7.6631) -> (-4.5115, -7.7876) centre (0, 0) ccw
  line L258 (-4.5628, -7.5393) -> (-4.7199, -7.6631)
  arc A257 (-4.5628, -7.5393) -> (-4.4769, -7.5906) centre (0, 0) ccw
  line L259 (-4.1575, -7.9822) -> (-4.1319, -7.7838)
  arc A258 (-4.3713, -7.8671) -> (-4.1575, -7.9822) centre (0, 0) ccw
  line L260 (-4.2199, -7.7364) -> (-4.3713, -7.8671)
  arc A259 (-4.2199, -7.7364) -> (-4.1319, -7.7838) centre (0, 0) ccw
  line L261 (-3.7952, -8.1607) -> (-3.7785, -7.9614)
  arc A260 (-4.014, -8.0553) -> (-3.7952, -8.1607) centre (0, 0) ccw
  line L262 (-3.8686, -7.918) -> (-4.014, -8.0553)
  arc A261 (-3.8686, -7.918) -> (-3.7785, -7.9614) centre (0, 0) ccw
  line L263 (-3.4253, -8.3227) -> (-3.4175, -8.1229)
  arc A262 (-3.6485, -8.2273) -> (-3.4253, -8.3227) centre (0, 0) ccw
  line L264 (-3.5095, -8.0836) -> (-3.6485, -8.2273)
  arc A263 (-3.5095, -8.0836) -> (-3.4175, -8.1229) centre (0, 0) ccw
  line L265 (-3.0484, -8.468) -> (-3.0496, -8.268)
  arc A264 (-3.2757, -8.3827) -> (-3.0484, -8.468) centre (0, 0) ccw
  line L266 (-3.1433, -8.2329) -> (-3.2757, -8.3827)
  arc A265 (-3.1433, -8.2329) -> (-3.0496, -8.268) centre (0, 0) ccw
  line L267 (-2.6654, -8.5962) -> (-2.6756, -8.3965)
  arc A266 (-2.8964, -8.5212) -> (-2.6654, -8.5962) centre (0, 0) ccw
  line L268 (-2.7707, -8.3656) -> (-2.8964, -8.5212)
  arc A267 (-2.7707, -8.3656) -> (-2.6756, -8.3965) centre (0, 0) ccw
  line L269 (-2.2771, -8.7072) -> (-2.2962, -8.5081)
  arc A268 (-2.5111, -8.6426) -> (-2.2771, -8.7072) centre (0, 0) ccw
  line L270 (-2.3926, -8.4815) -> (-2.5111, -8.6426)
  arc A269 (-2.3926, -8.4815) -> (-2.2962, -8.5081) centre (0, 0) ccw
  line L271 (-1.8842, -8.8006) -> (-1.9122, -8.6025)
  arc A270 (-2.1209, -8.7465) -> (-1.8842, -8.8006) centre (0, 0) ccw
  line L272 (-2.0097, -8.5803) -> (-2.1209, -8.7465)
  arc A271 (-2.0097, -8.5803) -> (-1.9122, -8.6025) centre (0, 0) ccw
  line L273 (-1.4874, -8.8762) -> (-1.5243, -8.6797)
  arc A272 (-1.7263, -8.8329) -> (-1.4874, -8.8762) centre (0, 0) ccw
  line L274 (-1.6227, -8.6618) -> (-1.7263, -8.8329)
  arc A273 (-1.6227, -8.6618) -> (-1.5243, -8.6797) centre (0, 0) ccw
  line L275 (-1.0877, -8.934) -> (-1.1334, -8.7393)
  arc A274 (-1.3283, -8.9014) -> (-1.0877, -8.934) centre (0, 0) ccw
  line L276 (-1.2325, -8.7259) -> (-1.3283, -8.9014)
  arc A275 (-1.2325, -8.7259) -> (-1.1334, -8.7393) centre (0, 0) ccw
  line L277 (-0.6858, -8.9738) -> (-0.7401, -8.7814)
  arc A276 (-0.9276, -8.9521) -> (-0.6858, -8.9738) centre (0, 0) ccw
  line L278 (-0.8397, -8.7724) -> (-0.9276, -8.9521)
  arc A277 (-0.8397, -8.7724) -> (-0.7401, -8.7814) centre (0, 0) ccw
  line L279 (-0.2825, -8.9956) -> (-0.3454, -8.8057)
  arc A278 (-0.525, -8.9847) -> (-0.2825, -8.9956) centre (0, 0) ccw
  line L280 (-0.4453, -8.8012) -> (-0.525, -8.9847)
  arc A279 (-0.4453, -8.8012) -> (-0.3454, -8.8057) centre (0, 0) ccw
  point P0 (0.3954, -8.8036)
  point P1 (0.7899, -8.777)
  point P2 (1.1829, -8.7327)
  point P3 (1.5735, -8.6709)
  point P4 (1.961, -8.5916)
  point P5 (2.3444, -8.4949)
  point P6 (2.7232, -8.3812)
  point P7 (3.0965, -8.2506)
  point P8 (3.4635, -8.1033)
  point P9 (3.8236, -7.9398)
  point P10 (4.176, -7.7602)
  point P11 (4.5199, -7.5651)
  point P12 (4.8548, -7.3547)
  point P13 (5.1799, -7.1295)
  point P14 (5.4945, -6.8899)
  point P15 (5.7981, -6.6364)
  point P16 (6.09, -6.3696)
  point P17 (6.3696, -6.09)
  point P18 (6.6364, -5.7981)
  point P19 (6.8899, -5.4945)
  point P20 (7.1295, -5.1799)
  point P21 (7.3547, -4.8548)
  point P22 (7.5651, -4.5199)
  point P23 (7.7602, -4.176)
  point P24 (7.9398, -3.8236)
  point P25 (8.1033, -3.4635)
  point P26 (8.2506, -3.0965)
  point P27 (8.3812, -2.7232)
  point P28 (8.4949, -2.3444)
  point P29 (8.5916, -1.961)
  point P30 (8.6709, -1.5735)
  point P31 (8.7327, -1.1829)
  point P32 (8.777, -0.7899)
  point P33 (8.8036, -0.3954)
  point P34 (8.8125, 0)
  point P35 (8.8036, 0.3954)
  point P36 (8.777, 0.7899)
  point P37 (8.7327, 1.1829)
  point P38 (8.6709, 1.5735)
  point P39 (8.5916, 1.961)
  point P40 (8.4949, 2.3444)
  point P41 (8.3812, 2.7232)
  point P42 (8.2506, 3.0965)
  point P43 (8.1033, 3.4635)
  point P44 (7.9398, 3.8236)
  point P45 (7.7602, 4.176)
  point P46 (7.5651, 4.5199)
  point P47 (7.3547, 4.8548)
  point P48 (7.1295, 5.1799)
  point P49 (6.8899, 5.4945)
  point P50 (6.6364, 5.7981)
  point P51 (6.3696, 6.09)
  point P52 (6.09, 6.3696)
  point P53 (5.7981, 6.6364)
  point P54 (5.4945, 6.8899)
  point P55 (5.1799, 7.1295)
  point P56 (4.8548, 7.3547)
  point P57 (4.5199, 7.5651)
  point P58 (4.176, 7.7602)
  point P59 (3.8236, 7.9398)
  point P60 (3.4635, 8.1033)
  point P61 (3.0965, 8.2506)
  point P62 (2.7232, 8.3812)
  point P63 (2.3444, 8.4949)
  point P64 (1.961, 8.5916)
  point P65 (1.5735, 8.6709)
  point P66 (1.1829, 8.7327)
  point P67 (0.7899, 8.777)
  point P68 (0.3954, 8.8036)
  point P69 (0, 8.8125)
  point P70 (-0.3954, 8.8036)
  point P71 (-0.7899, 8.777)
  point P72 (-1.1829, 8.7327)
  point P73 (-1.5735, 8.6709)
  point P74 (-1.961, 8.5916)
  point P75 (-2.3444, 8.4949)
  point P76 (-2.7232, 8.3812)
  point P77 (-3.0965, 8.2506)
  point P78 (-3.4635, 8.1033)
  point P79 (-3.8236, 7.9398)
  point P80 (-4.176, 7.7602)
  point P81 (-4.5199, 7.5651)
  point P82 (-4.8548, 7.3547)
  point P83 (-5.1799, 7.1295)
  point P84 (-5.4945, 6.8899)
  point P85 (-5.7981, 6.6364)
  point P86 (-6.09, 6.3696)
  point P87 (-6.3696, 6.09)
  point P88 (-6.6364, 5.7981)
  point P89 (-6.8899, 5.4945)
  point P90 (-7.1295, 5.1799)
  point P91 (-7.3547, 4.8548)
  point P92 (-7.5651, 4.5199)
  point P93 (-7.7602, 4.176)
  point P94 (-7.9398, 3.8236)
  point P95 (-8.1033, 3.4635)
  point P96 (-8.2506, 3.0965)
  point P97 (-8.3812, 2.7232)
  point P98 (-8.4949, 2.3444)
  point P99 (-8.5916, 1.961)
  point P100 (-8.6709, 1.5735)
  point P101 (-8.7327, 1.1829)
  point P102 (-8.777, 0.7899)
  point P103 (-8.8036, 0.3954)
  point P104 (-8.8125, 0)
  point P105 (-8.8036, -0.3954)
  point P106 (-8.777, -0.7899)
  point P107 (-8.7327, -1.1829)
  point P108 (-8.6709, -1.5735)
  point P109 (-8.5916, -1.961)
  point P110 (-8.4949, -2.3444)
  point P111 (-8.3812, -2.7232)
  point P112 (-8.2506, -3.0965)
  point P113 (-8.1033, -3.4635)
  point P114 (-7.9398, -3.8236)
  point P115 (-7.7602, -4.176)
  point P116 (-7.5651, -4.5199)
  point P117 (-7.3547, -4.8548)
  point P118 (-7.1295, -5.1799)
  point P119 (-6.8899, -5.4945)
  point P120 (-6.6364, -5.7981)
  point P121 (-6.3696, -6.09)
  point P122 (-6.09, -6.3696)
  point P123 (-5.7981, -6.6364)
  point P124 (-5.4945, -6.8899)
  point P125 (-5.1799, -7.1295)
  point P126 (-4.8548, -7.3547)
  point P127 (-4.5199, -7.5651)
  point P128 (-4.176, -7.7602)
  point P129 (-3.8236, -7.9398)
  point P130 (-3.4635, -8.1033)
  point P131 (-3.0965, -8.2506)
  point P132 (-2.7232, -8.3812)
  point P133 (-2.3444, -8.4949)
  point P134 (-1.961, -8.5916)
  point P135 (-1.5735, -8.6709)
  point P136 (-1.1829, -8.7327)
  point P137 (-0.7899, -8.777)
  point P138 (-0.3954, -8.8036)
  dimension "d9" = 18
  dimension "d11" = 0.2
  dimension "d12" = 0.2
  dimension "d13" = 0.1
  dimension "d15" = 0.05
  dimension "d16" = 17.625
  dimension "d19" = 360
  constraints: 700 point on circle, 562 end point, 280 centre point, 141 coincident, 1 vertical, 1541 other
  measures "d9" diameter of A0
  measures "d11" distance of L0.start L0.end
  measures "d12" distance of L1.start L1.end
  measures "d13" distance of L1.start L0.end
  measures "d15" distance from line of L2 L0.end
  measures "d16" diameter of A1
extrude "押し出し4" cut sketch "スケッチ4" against normal through all
equation "\"d12\" = d11"
